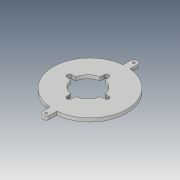
# Autodesk Inventor part: verticalThrusterCover
Saved by Autodesk Inventor 2018 (Build 220112000, 112)
## iProperties
Created: 2020-02-09
Part Number: verticalThrusterCover
Material: Generic
Document SubType Name: Modeling
Designer: anirudh
Density: 1 g/cm^3
Appearance: Default
Author: anirudh
Autodesk Inventor part; units mm, degrees
ref_plane "YZ Plane" through (0, 0, 0) normal (1, 0, 0) x (0, 1, 0)
ref_plane "XZ Plane" through (0, 0, 0) normal (0, 1, 0) x (-1, 0, 0)
ref_plane "XY Plane" through (0, 0, 0) normal (0, 0, 1) x (1, 0, 0)
sketch "Sketch1" plane through (0, 0, 0) normal (0, 1, 0) x (-1, 0, 0)
  circle A0 centre (0, -63.5) radius 1.75
  circle A1 centre (0, 63.5) radius 1.75
  circle A2 centre (0, -63.5) radius 1.75
  circle A3 centre (0, 63.5) radius 1.75
  arc A4 (5.08, 63.5) -> (-5.08, 63.5) centre (0, 63.5) ccw
  arc A5 (-5.08, -63.5) -> (5.08, -63.5) centre (0, -63.5) ccw
  line L0 (5.08, 63.5) -> (5.08, 53.0975)
  line L1 (5.08, -53.0975) -> (5.08, -63.5)
  line L2 (-5.08, -63.5) -> (-5.08, -53.0975)
  line L3 (-5.08, 53.0975) -> (-5.08, 63.5)
  arc A6 (-5.08, 53.0975) -> (-5.08, -53.0975) centre (0, 0) ccw
  arc A7 (5.08, -53.0975) -> (5.08, 53.0975) centre (0, 0) ccw
  arc A8 (-0.1848, -27.646) -> (6.1284, -27.646) centre (2.9718, -27.305) ccw
  line L4 (6.8199, -21.2443) -> (6.1284, -27.646)
  line L5 (-0.1848, -27.646) -> (-0.8763, -21.2443)
  line L6 (30.6178, -3.1566) -> (24.2161, -3.8481)
  line L7 (24.2161, 3.8481) -> (30.6178, 3.1566)
  arc A9 (30.6178, -3.1566) -> (30.6178, 3.1566) centre (30.2768, 0) ccw
  line L8 (6.1284, 27.646) -> (6.8199, 21.2443)
  line L9 (-0.8763, 21.2443) -> (-0.1848, 27.646)
  arc A10 (6.1284, 27.646) -> (-0.1848, 27.646) centre (2.9718, 27.305) ccw
  line L10 (-24.6742, 3.1566) -> (-18.2725, 3.8481)
  line L11 (-18.2725, -3.8481) -> (-24.6742, -3.1566)
  arc A11 (-24.6742, 3.1566) -> (-24.6742, -3.1566) centre (-24.3332, 0) ccw
  arc A12 (24.2161, 3.8481) -> (6.8199, 21.2443) centre (2.9718, 0) ccw
  arc A13 (-0.8763, 21.2443) -> (-18.2725, 3.8481) centre (2.9718, 0) ccw
  arc A14 (-18.2725, -3.8481) -> (-0.8763, -21.2443) centre (2.9718, 0) ccw
  arc A15 (6.8199, -21.2443) -> (24.2161, -3.8481) centre (2.9718, 0) ccw
  dimension "d34" = 360
  constraints: 24 end point, 24 point on circle, 16 centre point, 4 coincident, 4 vertical, 2 concentric, 33 other
extrude "Extrusion2" add sketch "Sketch1" along normal blind 5.08
body "Solid2"
